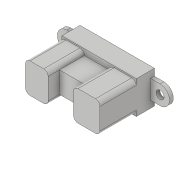
# Autodesk Inventor part: Sharp 2Y0A02
Saved by Autodesk Inventor 2018.3 (Build 223284000, 284)
## iProperties
Created: 2018-12-11
Part Number: Sharp 2Y0A02
Material: Generic
Document SubType Name: Modeling
Designer: aye06091
Mass: 7.04781 g
Surface Area: 29.3782 cm^2
Volume: 7.04781 cm^3
Density: 1 g/cm^3
Appearance: Default
Author: aye06091
Autodesk Inventor part; units mm, degrees
ref_plane "YZ Plane" through (0, 0, 0) normal (1, 0, 0) x (0, 1, 0)
ref_plane "XZ Plane" through (0, 0, 0) normal (0, 1, 0) x (-1, 0, 0)
sketch "Sketch1" plane through (0, 0, 0) normal (0, 0, 1) x (1, 0, 0)
  line L0 (0, 0) -> (29.5, 0)
  line L1 (29.5, 0) -> (29.5, -18.9)
  line L2 (29.5, -18.9) -> (0, -18.9)
  line L3 (0, -18.9) -> (0, 0)
  dimension "d0" = 29.5
  dimension "d1" = 18.9
  constraints: 8 end point, 2 parallel, 1 horizontal, 1 perpendicular
  measures "d0" distance of L0.start L0.end
  measures "d1" distance of L0.end L1.end
extrude "Extrusion1" add sketch "Sketch1" against normal blind 21.6
sketch "Sketch2" plane through (0, 0, 0) normal (0, 0, 1) x (1, 0, 0)
  line L0 (0, 0) -> (29.5, 0) projected
  line L1 (29.5, -18.9) -> (0, -18.9) projected
  line L2 (0, -18.9) -> (0, 0) projected
  line L3 (0, 0) -> (29.5, 0)
  line L4 (29.5, 0) -> (29.5, -13)
  line L5 (29.5, -13) -> (0, -13)
  line L6 (0, -13) -> (0, 0)
  line L7 (9.7099, -18.9) -> (19.8099, -18.9)
  line L8 (19.8099, -18.9) -> (19.8099, -13)
  line L9 (19.8099, -13) -> (9.7099, -13)
  line L10 (9.7099, -13) -> (9.7099, -18.9)
  line L11 (29.5, 0) -> (29.5, -18.9) projected
  dimension "d6" = 13
  dimension "d11" = 10.1
  dimension "d39" = 9.6901
  constraints: 16 end point, 4 parallel, 2 horizontal, 2 perpendicular, 2 point on line, 1 collinear
  measures "d6" distance between parallel lines of L5 L0
  measures "d11" distance between parallel lines of L8 L10
  measures "d39" distance between parallel lines of L11 L8
extrude "Extrusion2" cut sketch "Sketch2" against normal blind 21.6 contours L5 L10 L1 L2 | L11 L1 L8 L5
sketch "Sketch4" plane through (0, 0, 0) normal (0, 0, 1) x (1, 0, 0)
  line L0 (9.7099, -13) -> (9.7099, -18.9) projected
  line L1 (29.5, -18.9) -> (0, -18.9) projected
  line L2 (19.8099, -18.9) -> (19.8099, -13) projected
  line L3 (19.8099, -13) -> (29.5, -13) projected
  line L4 (29.5, 0) -> (29.5, -18.9) projected
  line L5 (0, 0) -> (29.5, 0) projected
  line L6 (0, -18.9) -> (0, 0) projected
  line L7 (0, -13) -> (9.7099, -13) projected
extrude "Extrusion3" cut sketch "Sketch4" against normal blind 14.4 contours L7 L6 L5 L4 L3 L2 L1 L0
sketch "Sketch5" plane through (0, 0, -14.4) normal (0, 0, 1) x (1, 0, 0)
  line L0 (29.5, 0) -> (29.5, -13) projected
  line L1 (0, 0) -> (29.5, 0) projected
  line L2 (0, -13) -> (0, 0) projected
  line L3 (0, -0.5461) -> (8.95, -0.5461)
  line L4 (8.95, -0.5461) -> (8.95, -12.4461)
  line L5 (8.95, -12.4461) -> (0, -12.4461)
  line L6 (0, -12.4461) -> (0, -0.5461)
  line L7 (19.05, -0.5461) -> (29.5, -0.5461)
  line L8 (29.5, -0.5461) -> (29.5, -12.4461)
  line L9 (29.5, -12.4461) -> (19.05, -12.4461)
  line L10 (19.05, -12.4461) -> (19.05, -0.5461)
  point P0 (33.25, -13)
  dimension "d22" = 8.95
  dimension "d23" = 10.45
  dimension "d24" = 11.9
  dimension "d25" = 11.9
  dimension "d26" = 0.5461
  dimension "d27" = 0.5461
  constraints: 16 end point, 4 parallel, 2 collinear, 2 horizontal, 2 perpendicular, 1 vertical, 1 other
  measures "d22" distance of L3.start L3.end
  measures "d23" distance of L7.start L7.end
  measures "d24" distance of L3.end L4.end
  measures "d25" distance of L9.end L7.start
  measures "d26" distance between parallel lines of L1 L3
  measures "d27" distance between parallel lines of L1 L7
extrude "Extrusion4" add sketch "Sketch5" along normal blind 14.4
fillet "Fillet1" radius 1.75 8 edges at (8.95, -0.5461, -7.2) (8.95, -12.4461, -7.2) (0, -0.5461, -7.2) (29.5, -0.5461, -7.2) (19.05, -0.5461, -7.2) (29.5, -12.4461, -7.2) (0, -12.4461, -7.2) (19.05, -12.4461, -7.2)
sketch "Sketch6" plane through (0, 0, -14.4) normal (0, 0, 1) x (1, 0, 0)
  line L0 (19.05, -10.6961) -> (19.05, -2.2961) projected
  line L1 (0, 0) -> (29.5, 0) projected
  line L2 (8.95, -2.2961) -> (8.95, -10.6961) projected
  line L3 (8.95, -2.2987) -> (19.05, -2.2987)
  line L4 (19.05, -2.2987) -> (19.05, -10.6987)
  line L5 (19.05, -10.6987) -> (8.95, -10.6987)
  line L6 (8.95, -10.6987) -> (8.95, -2.2987)
  dimension "d31" = 8.4
  dimension "d32" = 2.2987
  constraints: 8 end point, 2 parallel, 2 point on line, 1 horizontal, 1 perpendicular
  measures "d31" distance between parallel lines of L5 L3
  measures "d32" distance between parallel lines of L1 L3
extrude "Extrusion5" add sketch "Sketch6" along normal blind 9.9
sketch "Sketch8" plane through (0, 0, -21.6) normal (0, 0, -1) x (-1, 0, 0)
  line L0 (-9.7099, -18.9) -> (-9.7099, -13) projected
  line L1 (-9.7099, -13) -> (0, -13) projected
  line L2 (0, -13) -> (0, 0) projected
  line L3 (0, 0) -> (-29.5, 0) projected
  line L4 (-29.5, 0) -> (-29.5, -13) projected
  line L5 (-29.5, -13) -> (-19.8099, -13) projected
  line L6 (-19.8099, -13) -> (-19.8099, -18.9) projected
  line L7 (-19.8099, -18.9) -> (-9.7099, -18.9) projected
  circle A0 centre (-33.25, -6.5) radius 3.75
  circle A1 centre (-33.25, -6.5) radius 1.6
  circle A2 centre (3.75, -6.5) radius 3.75
  circle A3 centre (3.75, -6.5) radius 1.6
  line L8 (-33.25, -2.75) -> (-29.5, -2.75)
  line L9 (-33.25, -10.25) -> (-29.5, -10.25)
  line L10 (3.75, -10.25) -> (0, -10.25)
  line L11 (3.75, -2.75) -> (0, -2.75)
  dimension "d40" = 37
  dimension "d41" = 7.5
  dimension "d42" = 3.2
  dimension "d43" = 7.5
  dimension "d44" = 3.2
  dimension "d46" = 29.5
  constraints: 8 end point, 6 point on line, 4 centre point, 4 point on circle, 2 coincident, 2 perpendicular, 2 tangent, 1 horizontal
  measures "d40" distance of A2.centre A0.centre
  measures "d41" diameter of A0
  measures "d42" diameter of A1
  measures "d43" diameter of A2
  measures "d44" diameter of A3
  measures "d46" distance between parallel lines of L2 L4
extrude "Extrusion6" add sketch "Sketch8" against normal blind 1.5 contours L2 A2 L10 | L2 L11 A2 | A2 | L9 A0 L4 | A0 L8 L4 | A0
sketch "Sketch10" plane through (0, 0, -14.4) normal (0, 0, 1) x (1, 0, 0)
  line L0 (9.7099, -18.9) -> (9.7099, -13) projected
  line L1 (9.7099, -13) -> (19.8099, -13)
  line L2 (19.8099, -13) -> (19.8099, -18.9)
  line L3 (19.8099, -18.9) -> (9.7099, -18.9)
  line L4 (9.7099, -18.9) -> (9.7099, -13)
  point P0 (0, 0)
  constraints: 8 end point, 2 parallel, 1 horizontal, 1 perpendicular
extrude "Extrusion7" cut sketch "Sketch10" against normal blind 6
ref_plane "Work Plane5" through (0, 0, -18.3) normal (0, 0, -1) x (-1, 0, 0)
sketch "Sketch11" plane through (0, 0, -18.3) normal (0, 0, -1) x (-1, 0, 0)
  line L0 (-19.8099, -18.9) -> (-9.7099, -18.9) projected
  line L1 (-9.7099, -13) -> (-19.8099, -13)
  line L2 (-19.8099, -13) -> (-19.8099, -18.9)
  line L3 (-19.8099, -18.9) -> (-9.7099, -18.9)
  line L4 (-9.7099, -18.9) -> (-9.7099, -13)
  point P0 (0, 0)
  constraints: 8 end point, 2 parallel, 1 horizontal, 1 perpendicular
extrude "Extrusion8" add sketch "Sketch11" against normal blind 1.2
sketch "Sketch12" plane through (0, 0, -20.4) normal (0, 0, 1) x (1, 0, 0)
  line L0 (9.7099, -13) -> (0, -13) projected
  line L1 (19.8099, -13) -> (19.8099, -18.9) projected
  line L2 (9.7099, -13) -> (19.8099, -13)
  line L3 (19.8099, -13) -> (19.8099, -18.9)
  line L4 (19.8099, -18.9) -> (9.7099, -18.9)
  line L5 (9.7099, -18.9) -> (9.7099, -13)
  point P0 (0, 0)
  constraints: 8 end point, 2 parallel, 1 horizontal, 1 perpendicular
extrude "Extrusion9" cut sketch "Sketch12" against normal blind 1.2
body "Solid1"
